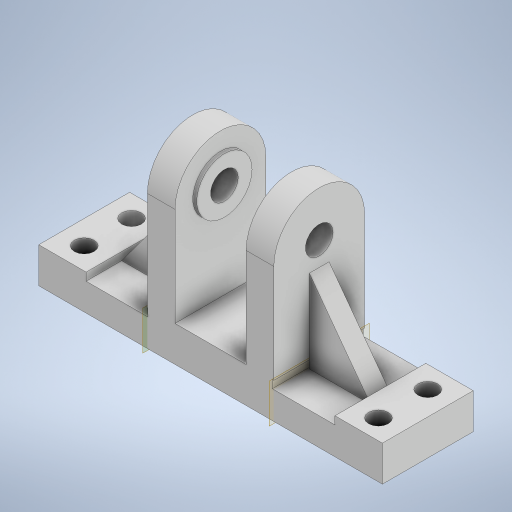
# Autodesk Inventor part: 5 - Part1
Saved by Autodesk Inventor 2024 (Build 280153000, 153)
## iProperties
Created: 2024-04-24
Part Number: 5 - Part1
Material: Generic
Document SubType Name: Modeling
Designer: Ricsi
Density: 1 g/cm^3
Appearance: Default
Author: Ricsi
Autodesk Inventor part; units mm, degrees
ref_plane "YZ Plane" through (0, 0, 0) normal (1, 0, 0) x (0, 1, 0)
ref_plane "XZ Plane" through (0, 0, 0) normal (0, 1, 0) x (-1, 0, 0)
ref_plane "XY Plane" through (0, 0, 0) normal (0, 0, 1) x (1, 0, 0)
sketch "Sketch1" plane through (0, 0, 0) normal (0, 1, 0) x (-1, 0, 0)
  line L0 (0, 9.3285) -> (174, 9.3285)
  line L1 (174, 9.3285) -> (174, 55.3285)
  line L2 (174, 55.3285) -> (0, 55.3285)
  line L3 (0, 55.3285) -> (0, 9.3285)
  circle A0 centre (12, 45.3285) radius 5
  circle A1 centre (162, 44.3285) radius 5
  circle A2 centre (162, 20.3285) radius 5
  circle A3 centre (12, 20.3285) radius 5
  point P0 (0, 0)
  dimension "d0" = 174
  dimension "d1" = 46
  dimension "d2" = 10
  dimension "d3" = 12
  dimension "d4" = 10
  dimension "d5" = 10
  dimension "d6" = 11
  dimension "d7" = 12
  dimension "d8" = 10
  dimension "d9" = 12
  dimension "d10" = 11
  dimension "d11" = 10
  dimension "d12" = 12
  dimension "d13" = 11
  constraints: 8 end point, 4 centre point, 2 parallel, 1 horizontal, 1 perpendicular
  measures "d0" distance of L2.end L1.end
  measures "d1" distance of L1.end L0.end
  measures "d2" diameter of A0
  measures "d3" distance from line of A0.centre L3
  measures "d4" distance from line of A0.centre L2
  measures "d5" diameter of A1
  measures "d6" distance from line of L2 A1.centre
  measures "d7" distance from line of L1 A1.centre
  measures "d8" diameter of A2
  measures "d9" distance from line of L1 A2.centre
  measures "d10" distance from line of L0 A2.centre
  measures "d11" diameter of A3
  measures "d12" distance from line of L3 A3.centre
  measures "d13" distance from line of L0 A3.centre
extrude "Extrusion1" add sketch "Sketch1" along normal blind 18
ref_plane "Work Plane1" through (-55, 0, 55.3285) normal (1, 0, 0) x (0, 0, -1)
sketch "Sketch2" plane through (-55, 0, 55.3285) normal (1, 0, 0) x (0, 0, -1)
  line L0 (46, 18) -> (0, 18) projected
  line L1 (0, 18) -> (0, 68)
  line L2 (46, 18) -> (46, 68)
  circle A0 centre (23, 68) radius 7
  arc A1 (46, 68) -> (0, 68) centre (23, 68) ccw
  point P0 (55.3285, 0)
  dimension "d17" = 50
  dimension "d18" = 50
  dimension "d20" = 14
  constraints: 4 end point, 2 centre point, 2 point on circle, 2 vertical, 1 tangent
  measures "d17" distance of L0.end L1.end
  measures "d18" distance of L0.start L2.end
  measures "d20" diameter of A0
extrude "Extrusion2" add sketch "Sketch2" against normal blind 14
ref_plane "Work Plane2" through (-119, 0, 9.3285) normal (-1, 0, 0) x (0, 0, 1)
sketch "Sketch3" plane through (-119, 0, 9.3285) normal (-1, 0, 0) x (0, 0, 1)
  line L0 (0, 0) -> (0, 18) projected
  line L1 (0, 18) -> (0, 68)
  circle A0 centre (23, 68) radius 7 projected
  circle A1 centre (23, 68) radius 7
  line L2 (46, 0) -> (46, 18) projected
  line L3 (46, 18) -> (46, 68) projected
  line L4 (46, 18) -> (46, 68)
  arc A2 (46, 68) -> (0, 68) centre (23, 68) ccw
  line L5 (0, 18) -> (46, 18)
  point P0 (-9.3285, 0)
  dimension "d24" = 50
  dimension "d26" = 50
  constraints: 6 end point, 2 centre point, 2 point on circle, 2 vertical, 1 coincident, 1 horizontal, 1 tangent
  measures "d24" distance of L0.end L1.end
  measures "d26" distance of L2.end L3.end
extrude "Extrusion3" add sketch "Sketch3" against normal blind 14
sketch "Sketch4" plane through (-105, 0, 9.3285) normal (1, 0, 0) x (0, 0, -1)
  line L0 (-46, 19.0772) -> (-46, 69.0772)
  circle A0 centre (-23, 68) radius 14
  point P0 (9.3285, 0)
  dimension "d31" = 28
  constraints: 2 end point, 1 centre point
  measures "d31" diameter of A0
extrude "Extrusion4" add sketch "Sketch4" along normal blind 2
sketch "Sketch5" plane through (-103, 68, 32.3285) normal (1, 0, 0) x (0, 0, -1)
  circle A0 centre (0, 0) radius 14 projected
  circle A1 centre (0, 0) radius 7
  point P0 (32.3285, -68)
  dimension "d34" = 14
  constraints: 1 centre point, 1 coincident
  measures "d34" diameter of A1
extrude "Extrusion5" cut sketch "Sketch5" against normal blind 50 contours A1
sketch "Sketch6" plane through (0, 18, 0) normal (0, 1, 0) x (1, 0, 0)
  line L0 (0.0001, -55.3285) -> (-23.9999, -55.3285)
  line L1 (-23.9999, -55.3285) -> (-23.9999, -9.3285)
  line L2 (0, -9.3285) -> (-174, -9.3285) projected
  line L3 (-55.709, -55.3285) -> (-23.9999, -55.3285)
  line L4 (-23.9999, -9.3285) -> (-55.709, -9.3285)
  line L5 (-55.709, -55.3285) -> (-55.709, -9.3285)
  line L6 (-174, -55.3285) -> (-150, -55.3285)
  line L7 (-150, -55.3285) -> (-150, -9.3285)
  line L8 (-150, -55.3285) -> (-118.7635, -55.3285)
  line L9 (-174, -55.3285) -> (0, -55.3285) projected
  line L10 (-118.7635, -9.3285) -> (-118.7635, -55.3285)
  line L11 (-118.7635, -9.3285) -> (-150, -9.3285)
  point P0 (0, 0)
  dimension "d37" = 24
  dimension "d38" = 24
  constraints: 20 end point, 5 point on line, 3 perpendicular, 1 collinear, 1 vertical
  measures "d37" distance of L0.start L0.end
  measures "d38" distance of L6.start L6.end
extrude "Extrusion6" cut sketch "Sketch6" against normal blind 4 contours L3 L5 L2 L1 | L8 L7 L2 L10
sketch "Sketch7" plane through (-55, 0, 55.3285) normal (1, 0, 0) x (0, 0, -1)
  line L0 (0, 18) -> (0, 68)
  line L1 (23, 56) -> (28, 56)
  line L2 (23, 56) -> (18, 56)
  line L3 (18, 56) -> (18, 14)
  line L4 (0, 14) -> (46, 14) projected
  line L5 (28, 56) -> (28, 14)
  line L6 (18, 14) -> (28, 14)
  point P0 (55.3285, 0)
  dimension "d45" = 5
  dimension "d46" = 5
  constraints: 12 end point, 2 horizontal, 2 point on line, 1 collinear, 1 parallel, 1 vertical
  measures "d45" distance of L1.start L2.end
  measures "d46" distance of L1.start L1.end
extrude "Extrusion7" add sketch "Sketch7" along normal blind 31
sketch "Sketch8" plane through (-55, 14, 37.3285) normal (0, 0, 1) x (1, 0, 0)
  line L0 (0, 4) -> (0, 42) projected
  line L1 (31, 42) -> (31, 0) projected
  line L2 (0, 42) -> (31, 0)
  line L3 (31, 0) -> (31, 42)
  line L4 (31, 42) -> (0, 42)
  point P0 (55, -14)
  constraints: 6 end point, 1 collinear, 1 perpendicular
extrude "Extrusion8" cut sketch "Sketch8" against normal blind 31
sketch "Sketch9" plane through (-119, 0, 9.3285) normal (-1, 0, 0) x (0, 0, 1)
  line L0 (0, 18) -> (0, 14) projected
  line L1 (0, 18) -> (0, 68)
  line L2 (28, 56) -> (18, 56) projected
  line L3 (23, 56) -> (28, 56)
  line L4 (23, 56) -> (18, 56)
  line L5 (18, 56) -> (18, 14)
  line L6 (0, 14) -> (46, 14) projected
  line L7 (28, 14) -> (28, 56)
  line L8 (28, 14) -> (18, 14)
  point P0 (-9.3285, 0)
  dimension "d55" = 5
  constraints: 12 end point, 3 collinear, 2 point on line, 2 vertical, 1 parallel
  measures "d55" distance of L3.start L2.end
extrude "Extrusion9" add sketch "Sketch9" along normal blind 31
sketch "Sketch10" plane through (-119, 14, 27.3285) normal (0, 0, -1) x (-1, 0, 0)
  line L0 (0, 42) -> (31, 0)
  line L1 (31, 0) -> (31, 42)
  line L2 (31, 42) -> (0, 42)
  point P0 (-119, -14)
  constraints: 6 end point, 1 perpendicular, 1 vertical
extrude "Extrusion10" cut sketch "Sketch10" against normal blind 31
sketch "Sketch11" plane through (-69, 0, 55.3285) normal (-1, 0, 0) x (0, 0, 1)
  circle A0 centre (-23, 68.0376) radius 14
  point P0 (-55.3285, 0)
  dimension "d60" = 28
  constraints: 1 centre point
  measures "d60" diameter of A0
extrude "Extrusion11" add sketch "Sketch11" along normal blind 2
sketch "Sketch12" plane through (-71, 68.0376, 32.3285) normal (-1, 0, 0) x (0, 0, 1)
  circle A0 centre (0, -0.0376) radius 7 projected
  circle A1 centre (0, -0.0376) radius 7
  point P0 (-32.3285, -68.0376)
  dimension "d63" = 14
  constraints: 1 centre point, 1 coincident
  measures "d63" diameter of A1
extrude "Extrusion12" cut sketch "Sketch12" against normal blind 50
body "Solid1"
